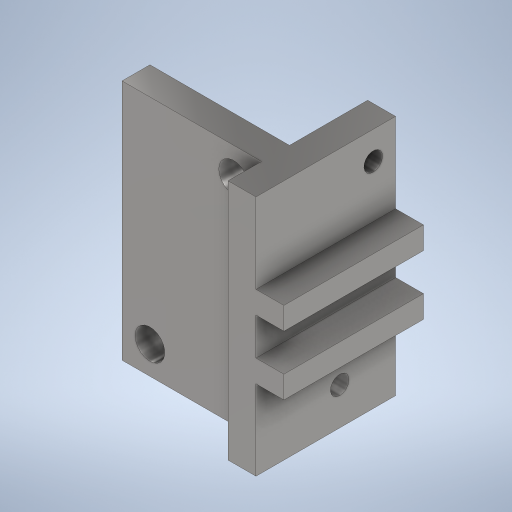
# Autodesk Inventor part: lager
Saved by Autodesk Inventor 2024 (Build 280153000, 153)
## iProperties
Created: 2024-02-02
Part Number: lager
Material: Edelstahl AISI 202
Document SubType Name: Modeling
Designer: ffogue
Density: 7.85472 g/cm^3
Appearance: Halbpoliert
Author: ffogue
Autodesk Inventor part; units mm, degrees
ref_plane "YZ Plane" through (0, 0, 0) normal (1, 0, 0) x (0, 1, 0)
ref_plane "XZ Plane" through (0, 0, 0) normal (0, 1, 0) x (-1, 0, 0)
sketch "Skizze1" plane through (0, 0, 0) normal (0, 0, 1) x (1, 0, 0)
  line L0 (0, 0) -> (15, 0)
  line L1 (15, 0) -> (15, 75)
  line L2 (15, 75) -> (0, 75)
  line L3 (0, 75) -> (0, 0)
  dimension "d0" = 15
  dimension "d1" = 75
  constraints: 8 end point, 2 parallel, 1 coincident, 1 horizontal, 1 perpendicular
  measures "d0" distance between parallel lines of L1 L3
  measures "d1" distance between parallel lines of L0 L2
extrude "Extrusion1" add sketch "Skizze1" along normal blind 130
sketch "Skizze2" plane through (0, 0, 0) normal (-1, 0, 0) x (0, 0, 1)
  line L0 (0, 0) -> (0, 75) projected
  line L1 (130, 0) -> (130, 75) projected
  line L2 (0, 33) -> (130, 33)
  line L3 (130, 33) -> (130, 18)
  line L4 (130, 18) -> (0, 18)
  line L5 (0, 18) -> (0, 33)
  line L6 (0, 0) -> (130, 0) projected
  point P0 (0, 18)
  dimension "d4" = 15
  dimension "d5" = 18
  constraints: 8 end point, 2 parallel, 2 point on line, 1 horizontal, 1 perpendicular
  measures "d4" distance between parallel lines of L4 L2
  measures "d5" distance between parallel lines of L6 L4
extrude "Extrusion2" add sketch "Skizze2" along normal blind 75 contours L0 L2 L1 L4
ref_plane "Arbeitsebene1" through (0, 0, 65) normal (0, 0, 1) x (1, 0, 0)
sketch "Skizze4" plane through (0, 0, 65) normal (0, 0, 1) x (1, 0, 0)
  line L0 (0, 75) -> (0, 33) projected
  line L1 (0, 75) -> (-42, 33)
  line L2 (0, 33) -> (-75, 33) projected
  point P0 (0, 0)
  dimension "d9" = 45
  constraints: 2 end point, 1 point on line
  measures "d9" angle of L2 L1
extrude "Extrusion3" add sketch "Skizze4" along normal mid plane 12
sketch "Skizze5" plane through (15, 0, 0) normal (1, 0, 0) x (0, 0, -1)
  line L0 (0, 75) -> (-130, 75) projected
  line L1 (-87, 75) -> (-75, 75)
  line L2 (-75, 75) -> (-75, 0)
  line L3 (-75, 0) -> (-87, 0)
  line L4 (-87, 0) -> (-87, 75)
  point P0 (0, 0)
  point P1 (-65, 75)
  dimension "d12" = 12
  dimension "d13" = 10
  dimension "d14" = 75
  constraints: 8 end point, 2 parallel, 1 horizontal, 1 midpoint, 1 perpendicular, 1 point on line
  measures "d12" distance between parallel lines of L2 L4
  measures "d13" distance from line of point (-65, 75) L2
  measures "d14" distance between parallel lines of L3 L0
extrude "Extrusion4" add sketch "Skizze5" along normal blind 15
mirror "Spiegeln1" about plane through (0, 0, 65) normal (0, 0, 1) of "Extrusion4"
sketch "Skizze6" plane through (0, 33, 0) normal (-1, 0, 0) x (0, 0, 1)
  line L0 (0, 42) -> (59, 42) projected
  line L1 (0, 42) -> (0, 0) projected
  point P0 (0, -33)
  point P1 (20, 12)
  dimension "d24" = 30
  dimension "d25" = 20
  measures "d24" distance from line of L0 point (20, 12)
  measures "d25" distance from line of point (20, 12) L1
hole "Bohrung1" at (0, 45, 20) direction (1, 0, 0) diameter 10 depth 15
sketch "Skizze7" plane through (0, 33, 130) normal (-1, 0, 0) x (0, 0, 1)
  line L0 (0, 0) -> (-130, 0) projected
  line L1 (0, 42) -> (0, 0) projected
  point P0 (-130, -33)
  point P1 (-15, 30)
  dimension "d33" = 30
  dimension "d34" = 15
  measures "d33" distance from line of L0 point (-15, 30)
  measures "d34" distance from line of L1 point (-15, 30)
hole "Bohrung" at (0, 63, 115) direction (1, 0, 0) diameter 10 end through all
sketch "Skizze8" plane through (-75, 33, 0) normal (0, 1, 0) x (1, 0, 0)
  line L0 (75, 0) -> (0, 0) projected
  line L1 (0, -130) -> (0, 0) projected
  point P0 (15, -15)
  dimension "d42" = 15
  dimension "d43" = 15
  measures "d42" distance from line of point (15, -15) L0
  measures "d43" distance from line of L1 point (15, -15)
hole "Bohrung3" at (-60, 33, 15) direction (0, -1, 0) diameter 16 end through all
sketch "Skizze9" plane through (-75, 33, 0) normal (0, 1, 0) x (1, 0, 0)
  line L0 (75, -130) -> (0, -130) projected
  line L1 (75, -71) -> (75, -130) projected
  point P0 (75, 0)
  point P1 (60, -115)
  dimension "d51" = 15
  dimension "d52" = 15
  measures "d51" distance from line of L0 point (60, -115)
  measures "d52" distance from line of L1 point (60, -115)
hole "Bohrung4" at (-15, 33, 115) direction (0, -1, 0) diameter 16 end through all
